Autodesk Fusion 360 part; units mm, degrees
(part 2 of 2)
sketch "Esquisse14" plane through (0, 0, 45) normal (0, 0, 1) x (-1, 0, 0)
  line L0 (-12, -12) -> (0, -12)
  line L1 (0, -12) -> (0, -3.5)
  arc A0 (-3.5, 0) -> (0, -3.5) centre (0, 0) ccw
  line L2 (-3.5, 0) -> (-12, 0)
  line L3 (-12, 0) -> (-12, -12)
  line L4 (0, 5.8) -> (-5.0229, 2.9)
  line L5 (-5.0229, 2.9) -> (-5.0229, -2.9)
  line L6 (-5.0229, -2.9) -> (0, -5.8)
  line L7 (0, -5.8) -> (5.0229, -2.9)
  line L8 (5.0229, -2.9) -> (5.0229, 2.9)
  line L9 (5.0229, 2.9) -> (0, 5.8)
  line L10 (0, 3.5) -> (0, 12)
  dimension "d13" = 5.8
  constraint coincident A0.centre origin
  constraint coincident L4.start L10
  measures "d13" distance of L4.start A0.centre
extrude "Extrusion26" cut sketch "Esquisse14" against normal blind 5 contours L1 A0 L2 L5 L6 | L1 A0 L2 L4 L5 L7 L8 L9 bodies 1 2 3 4
sketch "Esquisse15" plane through (0, 0, 25) normal (0, 0, -1) x (1, 0, 0)
  line L0 (12, 12) -> (0, 12)
  line L1 (0, 12) -> (0, 3.5)
  arc A0 (3.5, 0) -> (0, 3.5) centre (0, 0) ccw
  line L2 (3.5, 0) -> (12, 0)
  line L3 (12, 0) -> (12, 12)
  line L4 (0, 5.8) -> (-5.0229, 2.9)
  line L5 (-5.0229, 2.9) -> (-5.0229, -2.9)
  line L6 (-5.0229, -2.9) -> (0, -5.8)
  line L7 (0, -5.8) -> (5.0229, -2.9)
  line L8 (5.0229, -2.9) -> (5.0229, 2.9)
  line L9 (5.0229, 2.9) -> (0, 5.8)
  dimension "d76" = 5.8
  constraint coincident A0.centre origin
  measures "d76" distance of L4.start A0.centre
extrude "Extrusion27" cut sketch "Esquisse15" against normal blind 5 contours L1 A0 L2 L8 L9 | L1 A0 L2 L4 L5 L6 L7 L8 bodies 1 2 3 4
